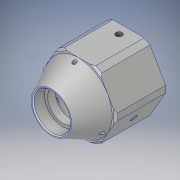
# Autodesk Inventor part: support_canon
Saved by Autodesk Inventor 2019 (Build 230136000, 136)
## iProperties
Created: 2019-03-26
Part Number: support_canon
Material: Aluminium 6061
Document SubType Name: Modeling
Designer: theor
Density: 2.7 g/cm^3
Appearance: Aluminium - Plat
Mass: 60.6569 g
Surface Area: 83.0197 cm^2
Volume: 22.4655 cm^3
Author: theor
Autodesk Inventor part; units mm, degrees
ref_plane "YZ Plane" through (0, 0, 0) normal (1, 0, 0) x (0, 1, 0)
ref_plane "XZ Plane" through (0, 0, 0) normal (0, 1, 0) x (-1, 0, 0)
ref_plane "XY Plane" through (0, 0, 0) normal (0, 0, 1) x (1, 0, 0)
sketch "Esquisse1" plane through (0, 0, 0) normal (1, 0, 0) x (0, 1, 0)
  line L0 (0, 0) -> (0, 17.727)
  line L1 (8, 30) -> (8, 34)
  line L2 (8, 30) -> (11, 30)
  line L3 (11, 30) -> (11, 0)
  line L4 (17.5, 26) -> (17.5, 0)
  line L5 (17.5, 0) -> (11, 0)
  line L6 (9.5, 40) -> (10.5, 40)
  line L7 (10.5, 40) -> (17.5, 26)
  line L8 (8, 34) -> (9.5, 34)
  line L9 (9.5, 40) -> (9.5, 34)
  dimension "d1" = 16
  dimension "d2" = 22
  dimension "d3" = 35
  dimension "d4" = 30
  dimension "d7" = 14
  dimension "d53" = 10
  dimension "d54" = 1.5
  dimension "d55" = 6
  dimension "d56" = 1
  constraints: 20 end point, 5 vertical, 4 horizontal, 1 horizontal alignment
  measures "d1" diameter of L1 L0
  measures "d2" diameter of L3 L0
  measures "d3" diameter of L4 L0
  measures "d4" distance of L2.end L3.end
  measures "d7" vertical distance of L6.end L4.start
  measures "d53" distance between parallel lines of L2 L6
  measures "d54" distance of L1.end L8.end
  measures "d55" distance of L6.start L8.end
  measures "d56" distance of L6.start L6.end
revolve "Révolution1" add sketch "Esquisse1" angle 360 about axis through (0, 0, 0) along (0, 0, 1)
sketch "Esquisse2" plane through (0, 0, 0) normal (0, 0, -1) x (-1, 0, 0)
  line L0 (10.1036, 17.5) -> (20.2073, 0)
  line L1 (20.2073, 0) -> (10.1036, -17.5)
  line L2 (10.1036, -17.5) -> (-10.1036, -17.5)
  line L3 (-10.1036, -17.5) -> (-20.2073, 0)
  line L4 (-20.2073, 0) -> (-10.1036, 17.5)
  line L5 (-10.1036, 17.5) -> (10.1036, 17.5)
  circle A0 centre (0, 0) radius 17.5 projected
  constraints: 12 end point, 1 coincident, 1 horizontal, 1 tangent, 13 other
extrude "Extrusion1" add sketch "Esquisse2" against normal blind 26 contours L0 A0 L5 | L0 L1 A0 | A0 L4 L5 | A0 L3 L4 | L1 L2 A0 | A0 L2 L3
chamfer "Chanfrein1" distance 1 angle 45 2 edges at (0, -11, 0) (0, -11, 30)
chamfer "Chanfrein2" distance 2 angle 45 6 edges at (10.1036, 17.5, 13) (20.2073, 0, 13) (10.1036, -17.5, 13) (-10.1036, -17.5, 13) (-20.2073, 0, 13) (-10.1036, 17.5, 13)
sketch "Esquisse3" plane through (-8.1036, -17.5, 0) normal (0, -1, 0) x (1, 0, 0)
  line L0 (0, 0) -> (16.2073, 0) projected
  line L1 (0, 26) -> (16.2073, 26) projected
  point P0 (8.1036, 0)
  point P1 (8.1036, 22)
  point P2 (8.1036, 8)
  point P3 (8.1036, 0)
  point P4 (8.1036, 0)
  point P5 (8.1036, 26)
  dimension "d17" = 8
  dimension "d26" = 14
  constraints: 2 midpoint, 2 vertical alignment
  measures "d17" distance of point (8.104, 8) point (8.104, 0)
  measures "d26" distance of point (8.104, 22) point (8.104, 8)
hole "Perçage1" at (0, -17.5, 22) at (0, -17.5, 8) direction (0, 1, 0) diameter 3.242 depth 4 tip angle 118 thread size "M4x0.7" class "6H" standard "ISO Metric profile"
sketch "Esquisse4" plane through (-8.1036, 17.5, 0) normal (0, 1, 0) x (1, 0, 0)
  point P0 (8.1036, 0)
  point P1 (8.1036, -5)
  dimension "d27" = 5
  constraints: 1 vertical alignment
  measures "d27" distance of point (8.104, 0) point (8.104, -5)
hole "Perçage2" at (0, 17.5, 5) direction (0, -1, 0) diameter 3.242 depth 4 thread size "M4x0.7" class "6H" standard "ISO Metric profile"
sketch "Esquisse5" plane through (0, 13.5, 5) normal (0, 1, 0) x (1, 0, 0)
  circle A0 centre (0, 0) radius 1.5
  circle A1 centre (0, 0) radius 1.621 projected
  point P0 (0, 5)
  dimension "d35" = 3
  constraints: 1 centre point, 1 coincident
  measures "d35" diameter of A0
extrude "Extrusion2" cut sketch "Esquisse5" against normal up to surface contours A0 round surface about axis through (0, 0, 15) along (0, 0, -1) radius 11 far side no
sketch "Esquisse6" plane through (-8.1036, 17.5, 0) normal (0, 1, 0) x (1, 0, 0)
  line L0 (16.2073, 0) -> (0, 0) projected
  line L1 (16.2073, -26) -> (0, -26) projected
  line L2 (18.6036, -40) -> (-2.3964, -40) projected
  point P0 (8.1036, 0)
  point P1 (8.1036, -28)
  point P2 (8.1036, 0)
  point P3 (8.1036, -26)
  dimension "d49" = 12
  constraints: 1 midpoint, 1 vertical alignment
  measures "d49" distance from line of L2 point (8.104, -28)
hole "Perçage3" at (0, 17.5, 28) direction (0, -1, 0) diameter 2 end up to surface
pattern_circular "Réseau circulaire1" count 3 over 360 about axis through (0, 0, -10) along (0, 0, 1) of "Perçage3"
chamfer "Chanfrein4" distance 0.5 angle 45 1 edges at (0, -9.5, 40)
chamfer "Chanfrein5" distance 1 angle 45 6 edges at (9.6036, 16.634, 26) (19.2073, 0, 26) (9.6036, -16.634, 26) (-9.6036, -16.634, 26) (-19.2073, 0, 26) (-9.6036, 16.634, 26)
sketch "Esquisse7" plane through (-19.2073, -1.7321, 0) normal (-0.8660254, -0.5, 0) x (0, 0, 1)
  line L0 (25, -16.2073) -> (0, -16.2073) projected
  point P0 (0, -8.1036)
  point P1 (12.5, -8.1036)
  point P2 (26, -8.1036)
  point P3 (12.5, -16.2073)
  constraints: 1 horizontal alignment, 1 midpoint, 1 vertical alignment
hole "Perçage4" at (-15.1554, -8.75, 12.5) direction (0.8660254, 0.5, 0) diameter 3.242 depth 4 tip angle 118 thread size "M4x0.7" class "6H" standard "ISO Metric profile"
mirror "Symétrie1" about plane through (0, 0, 0) normal (1, 0, 0) of "Perçage4"
